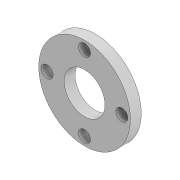
# Autodesk Inventor part: Part7
Saved by Autodesk Inventor 2020.5 (Build 245400000, 400)
## iProperties
Created: 2022-11-28
Part Number: Part7
Material: 一般
Document SubType Name: Modeling
Designer: Administrator
Density: 1 g/cm^3
Appearance: 既定
Author: Administrator
Autodesk Inventor part; units mm, degrees
ref_plane "YZ Plane" through (0, 0, 0) normal (1, 0, 0) x (0, 1, 0)
ref_plane "XZ Plane" through (0, 0, 0) normal (0, 1, 0) x (-1, 0, 0)
ref_plane "XY Plane" through (0, 0, 0) normal (0, 0, 1) x (1, 0, 0)
sketch "スケッチ1" plane through (0, 0, 0) normal (0, 0, 1) x (1, 0, 0)
  circle A0 centre (0, 0) radius 12.8 projected
  circle A1 centre (0, 11) radius 1.35 projected
  circle A2 centre (7.7782, 7.7782) radius 1.35 projected
  circle A3 centre (11, 0) radius 1.35 projected
  circle A4 centre (7.7782, -7.7782) radius 1.35 projected
  circle A5 centre (0, -11) radius 1.35 projected
  circle A6 centre (-7.7782, -7.7782) radius 1.35 projected
  circle A7 centre (-11, 0) radius 1.35 projected
  circle A8 centre (-7.7782, 7.7782) radius 1.35 projected
  circle A9 centre (0, 0) radius 5 projected
  circle A10 centre (0, 8) radius 1 projected
  circle A11 centre (-8, 0) radius 1 projected
  circle A12 centre (8, 0) radius 1 projected
  circle A13 centre (0, -8) radius 1 projected
  circle A14 centre (0, 0) radius 6
  circle A15 centre (0, 0) radius 13.5
  circle A16 centre (0, 11) radius 1.75
  circle A17 centre (-11, 0) radius 1.75
  circle A18 centre (0, -11) radius 1.75
  circle A19 centre (11, 0) radius 1.75
  point P0 (0, 0)
  dimension "d0" = 12
  dimension "d1" = 27
  dimension "d2" = 3.5
  dimension "d3" = 3.5
  dimension "d4" = 3.5
  dimension "d5" = 3.5
  constraints: 6 centre point, 6 coincident
  measures "d0" diameter of A14
  measures "d1" diameter of A15
  measures "d2" diameter of A16
  measures "d3" diameter of A17
  measures "d4" diameter of A18
  measures "d5" diameter of A19
extrude "押し出し1" add sketch "スケッチ1" along normal blind 3.2 contours A0 | A2 | A4 | A6 | A8 | A10 | A11 | A12 | A13 | A15
